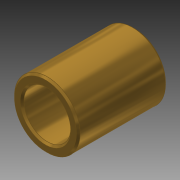
# Autodesk Inventor part: Rebuild Shooter NCDME075-0600 Cylinder Bushing
Saved by Autodesk Inventor 2014 SP1 (Build 180222100, 222)
## iProperties
Created: 2013-12-20
Part Number: Rebuild Shooter NCDME075-0600 Cylinder Bushing
Material: Brass, Soft Yellow
Document SubType Name: Modeling
Designer: Moses
Mass: 3.08068 g
Surface Area: 6.24204 cm^2
Volume: 0.363717 cm^3
Density: 8.47 g/cm^3
Appearance: Brass - Satin
Author: Moses
Autodesk Inventor part; units mm, degrees
ref_plane "YZ Plane" through (0, 0, 0) normal (1, 0, 0) x (0, 1, 0)
ref_plane "XZ Plane" through (0, 0, 0) normal (0, 1, 0) x (-1, 0, 0)
ref_plane "XY Plane" through (0, 0, 0) normal (0, 0, 1) x (1, 0, 0)
sketch "Sketch1" plane through (0, 0, 0) normal (0, 0, 1) x (1, 0, 0)
  circle A0 centre (0, 0) radius 4.445
  circle A1 centre (0, 0) radius 3.175
  dimension "d0" = 8.89
  dimension "d1" = 6.35
  constraints: 2 centre point, 2 coincident
  measures "d0" diameter of A0
  measures "d1" diameter of A1
extrude "Extrusion1" add sketch "Sketch1" along normal blind 12.065
chamfer "Chamfer1" distance 0.254 angle 45 4 edges at (-4.445, 0, 12.065) (-3.175, 0, 12.065) (-4.445, 0, 0) (-3.175, 0, 0)
body "Solid1"
